Autodesk Inventor part; units mm, degrees
(part 2 of 2)
sketch "Sketch9" plane through (0, 0, -97.79) normal (-1, 0, 0) x (0, 0, 1)
  line L0 (9.525, 8.4784) -> (80.645, 8.4784)
  line L1 (80.645, 8.4784) -> (80.645, 20)
  line L2 (80.645, 20) -> (9.525, 20)
  line L3 (9.525, 20) -> (9.525, 8.4784)
  line L4 (22.4663, 10.485) -> (10.5537, 10.485) projected
  line L5 (14.478, 19.365) -> (18.542, 19.365) projected
  line L6 (10.16, 12.4916) -> (10.16, 15.2856) projected
  line L7 (33.0517, 13.3762) -> (33.5217, 13.3762) projected
  line L8 (33.5217, 13.3762) -> (33.5217, 13.012) projected
  line L9 (33.5217, 13.012) -> (33.0517, 13.012) projected
  line L10 (33.0517, 13.012) -> (33.0517, 13.3762) projected
  line L11 (34.0677, 13.3762) -> (34.5377, 13.3762) projected
  line L12 (34.5377, 13.3762) -> (34.5377, 13.012) projected
  line L13 (34.5377, 13.012) -> (34.0677, 13.012) projected
  line L14 (34.0677, 13.012) -> (34.0677, 13.3762) projected
  line L15 (30.0037, 13.3762) -> (30.4737, 13.3762) projected
  line L16 (30.4737, 13.3762) -> (30.4737, 13.012) projected
  line L17 (30.4737, 13.012) -> (30.0037, 13.012) projected
  line L18 (30.0037, 13.012) -> (30.0037, 13.3762) projected
  line L19 (35.5537, 13.3762) -> (35.5537, 13.012) projected
  line L20 (35.5537, 13.012) -> (35.0837, 13.012) projected
  line L21 (35.0837, 13.012) -> (35.0837, 13.3762) projected
  line L22 (35.0837, 13.3762) -> (35.5537, 13.3762) projected
  line L23 (36.4363, 16.3016) -> (34.7983, 16.3016) projected
  line L24 (34.7983, 16.3016) -> (34.7983, 17.3176) projected
  line L25 (36.4363, 17.3176) -> (37.7063, 17.3176) projected
  line L26 (34.8996, 18.222) -> (34.8996, 17.3176) projected
  line L27 (33.782, 18.222) -> (34.8996, 18.222) projected
  line L28 (33.782, 19.365) -> (33.782, 18.222) projected
  line L29 (29.718, 19.365) -> (33.782, 19.365) projected
  line L30 (29.718, 18.222) -> (29.718, 19.365) projected
  line L31 (28.6004, 18.222) -> (29.718, 18.222) projected
  line L32 (28.6004, 17.3176) -> (28.6004, 18.222) projected
  line L33 (26.1617, 17.3176) -> (28.6004, 17.3176) projected
  line L34 (26.1617, 17.3176) -> (26.1617, 16.3016) projected
  line L35 (26.1617, 16.3016) -> (25.7937, 16.3016) projected
  line L36 (25.7937, 15.2856) -> (25.7937, 16.3016) projected
  line L37 (25.4, 15.2856) -> (25.7937, 15.2856) projected
  line L38 (25.4, 12.4916) -> (25.4, 15.2856) projected
  line L39 (25.7937, 12.4916) -> (25.4, 12.4916) projected
  line L40 (25.7937, 10.485) -> (25.7937, 12.4916) projected
  line L41 (37.7063, 10.485) -> (25.7937, 10.485) projected
  line L42 (37.7063, 12.4916) -> (37.7063, 10.485) projected
  line L43 (38.1, 12.4916) -> (37.7063, 12.4916) projected
  line L44 (38.1, 15.2856) -> (38.1, 12.4916) projected
  line L45 (37.7063, 15.2856) -> (38.1, 15.2856) projected
  line L46 (37.7063, 17.3176) -> (37.7063, 15.2856) projected
  line L47 (47.0217, 13.3762) -> (47.4917, 13.3762) projected
  line L48 (47.4917, 13.3762) -> (47.4917, 13.012) projected
  line L49 (47.4917, 13.012) -> (47.0217, 13.012) projected
  line L50 (47.0217, 13.012) -> (47.0217, 13.3762) projected
  line L51 (48.5077, 13.3762) -> (48.5077, 13.012) projected
  line L52 (48.5077, 13.012) -> (48.0377, 13.012) projected
  line L53 (48.0377, 13.012) -> (48.0377, 13.3762) projected
  line L54 (48.0377, 13.3762) -> (48.5077, 13.3762) projected
  line L55 (44.4437, 13.3762) -> (44.4437, 13.012) projected
  line L56 (44.4437, 13.012) -> (43.9737, 13.012) projected
  line L57 (43.9737, 13.012) -> (43.9737, 13.3762) projected
  line L58 (43.9737, 13.3762) -> (44.4437, 13.3762) projected
  line L59 (49.5237, 13.3762) -> (49.5237, 13.012) projected
  line L60 (49.5237, 13.012) -> (49.0537, 13.012) projected
  line L61 (49.0537, 13.012) -> (49.0537, 13.3762) projected
  line L62 (49.0537, 13.3762) -> (49.5237, 13.3762) projected
  line L63 (42.6717, 17.3176) -> (42.6717, 16.3016) projected
  line L64 (42.6717, 16.3016) -> (41.0337, 16.3016) projected
  line L65 (39.7637, 15.2856) -> (39.7637, 17.3176) projected
  line L66 (39.37, 15.2856) -> (39.7637, 15.2856) projected
  line L67 (39.37, 12.4916) -> (39.37, 15.2856) projected
  line L68 (39.7637, 12.4916) -> (39.37, 12.4916) projected
  line L69 (39.7637, 10.485) -> (39.7637, 12.4916) projected
  line L70 (51.6763, 10.485) -> (39.7637, 10.485) projected
  line L71 (51.6763, 12.4916) -> (51.6763, 10.485) projected
  line L72 (52.07, 12.4916) -> (51.6763, 12.4916) projected
  line L73 (52.07, 15.2856) -> (52.07, 12.4916) projected
  line L74 (51.6763, 15.2856) -> (52.07, 15.2856) projected
  line L75 (51.6763, 17.3176) -> (51.6763, 15.2856) projected
  line L76 (50.4063, 16.3016) -> (48.7683, 16.3016) projected
  line L77 (48.7683, 16.3016) -> (48.7683, 17.3176) projected
  line L78 (50.4063, 17.3176) -> (51.6763, 17.3176) projected
  line L79 (48.8696, 18.222) -> (48.8696, 17.3176) projected
  line L80 (47.752, 18.222) -> (48.8696, 18.222) projected
  line L81 (47.752, 19.365) -> (47.752, 18.222) projected
  line L82 (43.688, 19.365) -> (47.752, 19.365) projected
  line L83 (43.688, 18.222) -> (43.688, 19.365) projected
  line L84 (42.5704, 18.222) -> (43.688, 18.222) projected
  line L85 (42.5704, 17.3176) -> (42.5704, 18.222) projected
  line L86 (39.7637, 17.3176) -> (41.0337, 17.3176) projected
  line L87 (60.9917, 13.3762) -> (61.4617, 13.3762) projected
  line L88 (61.4617, 13.3762) -> (61.4617, 13.012) projected
  line L89 (61.4617, 13.012) -> (60.9917, 13.012) projected
  line L90 (60.9917, 13.012) -> (60.9917, 13.3762) projected
  line L91 (62.0077, 13.012) -> (62.0077, 13.3762) projected
  line L92 (62.0077, 13.3762) -> (62.4777, 13.3762) projected
  line L93 (62.4777, 13.3762) -> (62.4777, 13.012) projected
  line L94 (62.4777, 13.012) -> (62.0077, 13.012) projected
  line L95 (58.4137, 13.3762) -> (58.4137, 13.012) projected
  line L96 (58.4137, 13.012) -> (57.9437, 13.012) projected
  line L97 (57.9437, 13.012) -> (57.9437, 13.3762) projected
  line L98 (57.9437, 13.3762) -> (58.4137, 13.3762) projected
  line L99 (63.4937, 13.3762) -> (63.4937, 13.012) projected
  line L100 (63.4937, 13.012) -> (63.0237, 13.012) projected
  line L101 (63.0237, 13.012) -> (63.0237, 13.3762) projected
  line L102 (63.0237, 13.3762) -> (63.4937, 13.3762) projected
  line L103 (65.6463, 16.3016) -> (65.2783, 16.3016) projected
  line L104 (65.2783, 16.3016) -> (65.2783, 17.3176) projected
  line L105 (62.8396, 17.3176) -> (65.2783, 17.3176) projected
  line L106 (62.8396, 18.222) -> (62.8396, 17.3176) projected
  line L107 (61.722, 18.222) -> (62.8396, 18.222) projected
  line L108 (61.722, 19.365) -> (61.722, 18.222) projected
  line L109 (57.658, 19.365) -> (61.722, 19.365) projected
  line L110 (57.658, 18.222) -> (57.658, 19.365) projected
  line L111 (56.5404, 18.222) -> (57.658, 18.222) projected
  line L112 (56.5404, 17.3176) -> (56.5404, 18.222) projected
  line L113 (53.7337, 17.3176) -> (55.0037, 17.3176) projected
  line L114 (56.6417, 17.3176) -> (56.6417, 16.3016) projected
  line L115 (56.6417, 16.3016) -> (55.0037, 16.3016) projected
  line L116 (53.7337, 15.2856) -> (53.7337, 17.3176) projected
  line L117 (53.34, 15.2856) -> (53.7337, 15.2856) projected
  line L118 (53.34, 12.4916) -> (53.34, 15.2856) projected
  line L119 (53.7337, 12.4916) -> (53.34, 12.4916) projected
  line L120 (53.7337, 10.485) -> (53.7337, 12.4916) projected
  line L121 (65.6463, 10.485) -> (53.7337, 10.485) projected
  line L122 (65.6463, 12.4916) -> (65.6463, 10.485) projected
  line L123 (66.04, 12.4916) -> (65.6463, 12.4916) projected
  line L124 (66.04, 15.2856) -> (66.04, 12.4916) projected
  line L125 (65.6463, 15.2856) -> (66.04, 15.2856) projected
  line L126 (65.6463, 16.3016) -> (65.6463, 15.2856) projected
  line L127 (77.4637, 13.012) -> (76.9937, 13.012) projected
  line L128 (76.9937, 13.012) -> (76.9937, 13.3762) projected
  line L129 (76.9937, 13.3762) -> (77.4637, 13.3762) projected
  line L130 (77.4637, 13.3762) -> (77.4637, 13.012) projected
  line L131 (76.4477, 13.012) -> (75.9777, 13.012) projected
  line L132 (75.9777, 13.012) -> (75.9777, 13.3762) projected
  line L133 (75.9777, 13.3762) -> (76.4477, 13.3762) projected
  line L134 (76.4477, 13.3762) -> (76.4477, 13.012) projected
  line L135 (72.3837, 13.3762) -> (72.3837, 13.012) projected
  line L136 (72.3837, 13.012) -> (71.9137, 13.012) projected
  line L137 (71.9137, 13.012) -> (71.9137, 13.3762) projected
  line L138 (71.9137, 13.3762) -> (72.3837, 13.3762) projected
  line L139 (75.4317, 13.3762) -> (75.4317, 13.012) projected
  line L140 (75.4317, 13.012) -> (74.9617, 13.012) projected
  line L141 (74.9617, 13.012) -> (74.9617, 13.3762) projected
  line L142 (74.9617, 13.3762) -> (75.4317, 13.3762) projected
  line L143 (70.6117, 17.3176) -> (70.6117, 16.3016) projected
  line L144 (70.6117, 16.3016) -> (68.9737, 16.3016) projected
  line L145 (79.6163, 16.3016) -> (79.2483, 16.3016) projected
  line L146 (79.2483, 16.3016) -> (79.2483, 17.3176) projected
  line L147 (19.0817, 13.012) -> (19.0817, 13.3762) projected
  line L148 (19.0817, 13.3762) -> (19.5517, 13.3762) projected
  line L149 (19.5517, 13.3762) -> (19.5517, 13.012) projected
  line L150 (19.5517, 13.012) -> (19.0817, 13.012) projected
  line L151 (20.0977, 13.012) -> (20.0977, 13.3762) projected
  line L152 (20.0977, 13.3762) -> (20.5677, 13.3762) projected
  line L153 (20.5677, 13.3762) -> (20.5677, 13.012) projected
  line L154 (20.5677, 13.012) -> (20.0977, 13.012) projected
  line L155 (16.0337, 13.012) -> (16.0337, 13.3762) projected
  line L156 (16.0337, 13.3762) -> (16.5037, 13.3762) projected
  line L157 (16.5037, 13.3762) -> (16.5037, 13.012) projected
  line L158 (16.5037, 13.012) -> (16.0337, 13.012) projected
  line L159 (21.1137, 13.012) -> (21.1137, 13.3762) projected
  line L160 (21.1137, 13.3762) -> (21.5837, 13.3762) projected
  line L161 (21.5837, 13.3762) -> (21.5837, 13.012) projected
  line L162 (21.5837, 13.012) -> (21.1137, 13.012) projected
  line L163 (12.1917, 17.3176) -> (12.1917, 16.3016) projected
  line L164 (12.1917, 16.3016) -> (10.5537, 16.3016) projected
  line L165 (10.5537, 15.2856) -> (10.5537, 16.3016) projected
  line L166 (10.16, 15.2856) -> (10.5537, 15.2856) projected
  line L167 (10.16, 12.4916) -> (10.16, 15.2856) projected
  line L168 (10.5537, 12.4916) -> (10.16, 12.4916) projected
  line L169 (10.5537, 10.485) -> (10.5537, 12.4916) projected
  line L170 (22.4663, 10.485) -> (10.5537, 10.485) projected
  line L171 (22.4663, 12.4916) -> (22.4663, 10.485) projected
  line L172 (22.86, 12.4916) -> (22.4663, 12.4916) projected
  line L173 (22.86, 15.2856) -> (22.86, 12.4916) projected
  line L174 (22.4663, 15.2856) -> (22.86, 15.2856) projected
  line L175 (22.4663, 16.3016) -> (22.4663, 15.2856) projected
  line L176 (22.4663, 16.3016) -> (20.8283, 16.3016) projected
  line L177 (20.8283, 16.3016) -> (20.8283, 17.3176) projected
  line L178 (19.6596, 17.3176) -> (20.8283, 17.3176) projected
  line L179 (19.6596, 18.222) -> (19.6596, 17.3176) projected
  line L180 (18.542, 18.222) -> (19.6596, 18.222) projected
  line L181 (18.542, 19.365) -> (18.542, 18.222) projected
  line L182 (14.478, 19.365) -> (18.542, 19.365) projected
  line L183 (14.478, 18.222) -> (14.478, 19.365) projected
  line L184 (13.3604, 18.222) -> (14.478, 18.222) projected
  line L185 (13.3604, 17.3176) -> (13.3604, 18.222) projected
  line L186 (12.1917, 17.3176) -> (13.3604, 17.3176) projected
  line L187 (10.5537, 16.3016) -> (10.5537, 17.3176) projected
  line L188 (10.5537, 16.3016) -> (12.1917, 16.3016) projected
  line L189 (12.1917, 16.3016) -> (12.1917, 17.3176) projected
  line L190 (10.5537, 17.3176) -> (12.1917, 17.3176) projected
  line L191 (20.8283, 17.3176) -> (22.4663, 17.3176) projected
  line L192 (20.8283, 17.3176) -> (20.8283, 16.3016) projected
  line L193 (20.8283, 16.3016) -> (22.4663, 16.3016) projected
  line L194 (22.4663, 17.3176) -> (22.4663, 16.3016) projected
  line L195 (25.7937, 16.3016) -> (26.1617, 16.3016) projected
  line L196 (26.1617, 16.3016) -> (26.1617, 17.3176) projected
  line L197 (25.7937, 17.3176) -> (26.1617, 17.3176) projected
  line L198 (25.7937, 16.3016) -> (25.7937, 17.3176) projected
  line L199 (34.8996, 17.3176) -> (36.4363, 17.3176) projected
  line L200 (34.7983, 17.3176) -> (34.7983, 16.3016) projected
  line L201 (34.7983, 16.3016) -> (36.4363, 16.3016) projected
  line L202 (42.6717, 16.3016) -> (42.6717, 17.3176) projected
  line L203 (41.0337, 17.3176) -> (42.5704, 17.3176) projected
  line L204 (41.0337, 16.3016) -> (42.6717, 16.3016) projected
  line L205 (48.8696, 17.3176) -> (50.4063, 17.3176) projected
  line L206 (48.7683, 17.3176) -> (48.7683, 16.3016) projected
  line L207 (48.7683, 16.3016) -> (50.4063, 16.3016) projected
  line L208 (56.6417, 16.3016) -> (56.6417, 17.3176) projected
  line L209 (55.0037, 17.3176) -> (56.5404, 17.3176) projected
  line L210 (55.0037, 16.3016) -> (56.6417, 16.3016) projected
  line L211 (65.2783, 17.3176) -> (65.6463, 17.3176) projected
  line L212 (65.2783, 17.3176) -> (65.2783, 16.3016) projected
  line L213 (65.2783, 16.3016) -> (65.6463, 16.3016) projected
  line L214 (65.6463, 17.3176) -> (65.6463, 16.3016) projected
  line L215 (68.9737, 16.3016) -> (70.6117, 16.3016) projected
  line L216 (70.6117, 16.3016) -> (70.6117, 17.3176) projected
  line L217 (79.2483, 17.3176) -> (79.2483, 16.3016) projected
  line L218 (79.2483, 16.3016) -> (79.6163, 16.3016) projected
  line L219 (56.6417, 17.3176) -> (56.5404, 17.3176) projected
  line L220 (55.0037, 17.3176) -> (55.0037, 16.3016) projected
  line L221 (50.4063, 16.3016) -> (50.4063, 17.3176) projected
  line L222 (48.8696, 17.3176) -> (48.7683, 17.3176) projected
  line L223 (42.6717, 17.3176) -> (42.5704, 17.3176) projected
  line L224 (41.0337, 17.3176) -> (41.0337, 16.3016) projected
  line L225 (36.4363, 16.3016) -> (36.4363, 17.3176) projected
  line L226 (34.8996, 17.3176) -> (34.7983, 17.3176) projected
  line L227 (56.5404, 17.3176) -> (56.6417, 17.3176) projected
  line L228 (55.0037, 16.3016) -> (55.0037, 17.3176) projected
  line L229 (41.0337, 16.3016) -> (41.0337, 17.3176) projected
  line L230 (50.4063, 17.3176) -> (50.4063, 16.3016) projected
  line L231 (48.7683, 17.3176) -> (48.8696, 17.3176) projected
  line L232 (42.5704, 17.3176) -> (42.6717, 17.3176) projected
  line L233 (36.4363, 17.3176) -> (36.4363, 16.3016) projected
  line L234 (34.7983, 17.3176) -> (34.8996, 17.3176) projected
  line L235 (79.6163, 17.3176) -> (79.6163, 16.3016) projected
  line L236 (79.2483, 17.3176) -> (79.6163, 17.3176) projected
  line L237 (70.6117, 17.3176) -> (70.5104, 17.3176) projected
  line L238 (68.9737, 17.3176) -> (70.5104, 17.3176) projected
  line L239 (68.9737, 17.3176) -> (68.9737, 16.3016) projected
  line L240 (68.9737, 16.3016) -> (68.9737, 17.3176) projected
  line L241 (67.7037, 17.3176) -> (68.9737, 17.3176) projected
  line L242 (67.7037, 15.2856) -> (67.7037, 17.3176) projected
  line L243 (67.31, 15.2856) -> (67.7037, 15.2856) projected
  line L244 (67.31, 12.4916) -> (67.31, 15.2856) projected
  line L245 (67.7037, 12.4916) -> (67.31, 12.4916) projected
  line L246 (67.7037, 10.485) -> (67.7037, 12.4916) projected
  line L247 (79.6163, 10.485) -> (67.7037, 10.485) projected
  line L248 (79.6163, 12.4916) -> (79.6163, 10.485) projected
  line L249 (80.01, 12.4916) -> (79.6163, 12.4916) projected
  line L250 (80.01, 15.2856) -> (80.01, 12.4916) projected
  line L251 (79.6163, 15.2856) -> (80.01, 15.2856) projected
  line L252 (79.6163, 16.3016) -> (79.6163, 15.2856) projected
  line L253 (76.8096, 17.3176) -> (79.2483, 17.3176) projected
  line L254 (76.8096, 18.222) -> (76.8096, 17.3176) projected
  line L255 (75.692, 18.222) -> (76.8096, 18.222) projected
  line L256 (75.692, 19.365) -> (75.692, 18.222) projected
  line L257 (71.628, 19.365) -> (75.692, 19.365) projected
  line L258 (71.628, 18.222) -> (71.628, 19.365) projected
  line L259 (70.5104, 18.222) -> (71.628, 18.222) projected
  line L260 (70.5104, 17.3176) -> (70.5104, 18.222) projected
  line L261 (70.5104, 17.3176) -> (70.6117, 17.3176) projected
  point P0 (97.79, 0)
  point P1 (65.6463, 16.3016)
  point P2 (25.7937, 16.3016)
  point P3 (55.3717, 17.3176)
  point P4 (50.0383, 17.3176)
  point P5 (41.4017, 17.3176)
  point P6 (41.4017, 17.3176)
  point P7 (39.7637, 16.3016)
  point P8 (36.0683, 17.3176)
  point P9 (25.7937, 16.3016)
  point P10 (25.7937, 16.3016)
  dimension "d61" = 2.0066
  dimension "d62" = 0.635
  dimension "d63" = 0.635
  dimension "d100" = 0.635
  constraints: 8 end point, 2 parallel, 1 horizontal, 1 perpendicular
  measures "d61" distance between parallel lines of L0 L4
  measures "d62" distance between parallel lines of L5 L2
  measures "d63" distance between parallel lines of L3 L6
  measures "d100" distance between parallel lines of L1 L250
extrude "Extrusion5" add sketch "Sketch9" along normal blind 0.0508 contours L3 L2 L1 L0
sketch "Sketch10" plane through (0, 22.86, 0) normal (0, 1, 0) x (1, 0, 0)
  arc A0 (6.35, 104.14) -> (0, 97.79) centre (6.35, 97.79) ccw projected
  line L0 (0, 97.79) -> (0, 6.35) projected
  arc A1 (0, 6.35) -> (6.35, 0) centre (6.35, 6.35) ccw projected
  line L1 (6.35, 0) -> (64.77, 0) projected
  arc A2 (64.77, 0) -> (71.12, 6.35) centre (64.77, 6.35) ccw projected
  line L2 (71.12, 6.35) -> (71.12, 97.79) projected
  arc A3 (71.12, 97.79) -> (64.77, 104.14) centre (64.77, 97.79) ccw projected
  line L3 (64.77, 104.14) -> (6.35, 104.14) projected
  line L4 (67.31, 97.79) -> (67.31, 6.35)
  arc A4 (64.77, 3.81) -> (67.31, 6.35) centre (64.77, 6.35) ccw
  line L5 (64.77, 3.81) -> (6.35, 3.81)
  arc A5 (3.81, 6.35) -> (6.35, 3.81) centre (6.35, 6.35) ccw
  line L6 (3.81, 6.35) -> (3.81, 97.79)
  arc A6 (6.35, 100.33) -> (3.81, 97.79) centre (6.35, 97.79) ccw
  line L7 (6.35, 100.33) -> (64.77, 100.33)
  arc A7 (67.31, 97.79) -> (64.77, 100.33) centre (64.77, 97.79) ccw
  point P0 (0, 0)
  dimension "d67" = 3.81
  constraints: 8 end point, 8 point on circle, 4 centre point, 7 other
  measures "d67" distance between parallel lines of L2 L4
extrude "Extrusion6" cut sketch "Sketch10" against normal blind 0.0254 contours L4 A4 L5 A5 L6 A6 L7 A7
sketch "Sketch11" plane through (0, 22.8346, 0) normal (0, 1, 0) x (1, 0, 0)
  line L0 (54.2098, 8.4494) -> (54.2098, 27.4994) construction
  line L1 (54.2098, 27.4994) -> (62.0584, 27.4994) construction
  line L2 (62.0584, 27.4994) -> (62.0584, 8.4494) construction
  line L3 (62.0584, 8.4494) -> (54.2098, 8.4494) construction
  point P0 (0, 0)
  dimension "d71" = 19.05
  constraints: 1 vertical, 2 other
  measures "d71" distance of L0.start L0.end
decal "Decal1"
sketch "Sketch12" plane through (0, 22.8346, 0) normal (0, 1, 0) x (1, 0, 0)
  arc A0 (3.81, 6.35) -> (6.35, 3.81) centre (6.35, 6.35) ccw projected
  line L0 (64.77, 3.81) -> (6.35, 3.81) projected
  arc A1 (64.77, 3.81) -> (67.31, 6.35) centre (64.77, 6.35) ccw projected
  line L1 (67.31, 97.79) -> (67.31, 6.35) projected
  arc A2 (67.31, 97.79) -> (64.77, 100.33) centre (64.77, 97.79) ccw projected
  line L2 (6.35, 100.33) -> (64.77, 100.33) projected
  arc A3 (6.35, 100.33) -> (3.81, 97.79) centre (6.35, 97.79) ccw projected
  line L3 (3.81, 6.35) -> (3.81, 97.79) projected
  arc A4 (67.564, 97.79) -> (64.77, 100.584) centre (64.77, 97.79) ccw
  line L4 (67.564, 97.79) -> (67.564, 6.35)
  arc A5 (64.77, 3.556) -> (67.564, 6.35) centre (64.77, 6.35) ccw
  line L5 (64.77, 3.556) -> (6.35, 3.556)
  arc A6 (3.556, 6.35) -> (6.35, 3.556) centre (6.35, 6.35) ccw
  line L6 (3.556, 6.35) -> (3.556, 97.79)
  arc A7 (6.35, 100.584) -> (3.556, 97.79) centre (6.35, 97.79) ccw
  line L7 (6.35, 100.584) -> (64.77, 100.584)
  point P0 (0, 0)
  dimension "d95" = 0.254
  constraints: 8 end point, 8 point on circle, 4 centre point, 7 other
  measures "d95" distance between parallel lines of L2 L7
extrude "Extrusion7" cut sketch "Sketch12" along normal mid plane 2.54
sketch "Sketch13" plane through (-0.0508, 0, -97.79) normal (-1, 0, 0) x (0, 0, 1)
  line L0 (22.86, 15.2856) -> (22.86, 12.4916) construction
  line L1 (22.86, 13.8886) -> (25.4, 13.8886) construction
  line L2 (25.4, 12.4916) -> (25.4, 15.2856) construction
  line L3 (9.525, 8.4784) -> (80.645, 8.4784) projected
  line L4 (24.1287, 19.2988) -> (24.1313, 19.2988) construction
  line L5 (24.1313, 20) -> (24.1313, 8.4784)
  line L6 (24.1313, 8.4784) -> (24.1287, 8.4784)
  line L7 (24.1287, 8.4784) -> (24.1287, 19.2988)
  line L8 (24.1287, 19.2988) -> (24.1313, 8.4784) construction
  line L9 (24.1313, 19.2988) -> (24.1287, 8.4784) construction
  line L10 (80.645, 20) -> (9.525, 20) projected
  line L11 (24.1313, 20) -> (24.1287, 20)
  line L12 (9.525, 20) -> (80.645, 20) projected
  line L13 (24.1287, 20) -> (24.1287, 19.2988)
  point P0 (97.79, 0)
  point P1 (24.13, 13.8886)
  dimension "d101" = 0.0025
  dimension "d104" = 0.0025
  constraints: 18 end point, 5 midpoint, 4 point on line, 2 parallel, 1 horizontal, 1 perpendicular
  measures "d101" distance of L5.end L6.end
  measures "d104" distance of L5.start L11.end
extrude "Extrusion8" add sketch "Sketch13" along normal blind 0.0003
sketch "Sketch15" plane through (0, 0, -97.79) normal (-1, 0, 0) x (0, 0, 1)
  line L0 (12.3435, 8.3954) -> (74.9302, 8.3954) construction
  line L1 (74.9302, 8.3954) -> (74.9302, 4.0491) construction
  line L2 (74.9302, 4.0491) -> (12.3435, 4.0491) construction
  line L3 (12.3435, 4.0491) -> (12.3435, 8.3954) construction
  point P0 (97.79, 0)
  constraints: 2 other
decal "Decal2"
sketch "Sketch17" plane through (0, 22.8346, 0) normal (0, 1, 0) x (1, 0, 0)
  line L0 (57.4552, 71.792) -> (57.4552, 81.8973) construction
  line L1 (57.4552, 81.8973) -> (59.3308, 81.8973) construction
  line L2 (59.3308, 81.8973) -> (59.3308, 71.792) construction
  line L3 (59.3308, 71.792) -> (57.4552, 71.792) construction
  dimension "d1" = 104.14
  constraints: 2 other
sketch "Sketch18" plane through (0, 22.8346, 0) normal (0, 1, 0) x (1, 0, 0)
  line L0 (56.7248, 88.513) -> (56.7248, 91.5064) construction
  line L1 (56.7248, 91.5064) -> (59.7183, 91.5064) construction
  line L2 (59.7183, 91.5064) -> (59.7183, 88.513) construction
  line L3 (59.7183, 88.513) -> (56.7248, 88.513) construction
  point P0 (0, 0)
  constraints: 2 other
decal "Decal3"
sketch "Sketch20" plane through (0, 22.8346, 0) normal (0, 1, 0) x (1, 0, 0)
  circle A0 centre (58.1933, 86.2143) radius 0.508
  point P0 (0, 0)
  dimension "d261" = 1.016
  constraints: 1 centre point
  measures "d261" diameter of A0
extrude "Extrusion9" add sketch "Sketch20" along normal blind 0.0508
equation "\"d21\" = -0.5 * d19 + 0.5 * d20"
equation "\"d94\" = -0.25 * d23 + 0.25 * d22"
equation "\"d34\" = 0.5 * d33"
equation "\"d40\" = d39"
equation "\"d48\" = 0.5 * d37"
equation "\"d49\" = 0.5 * d38"
equation "\"d19\" = 71.12"
body "Solid1"
